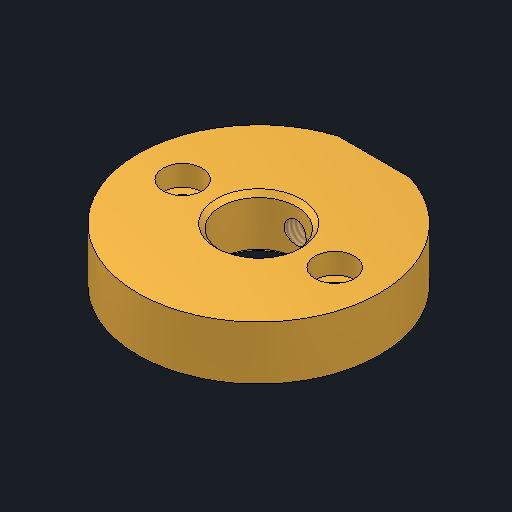
# Autodesk Inventor part: KN-00-02-12
Saved by Autodesk Inventor 2025.2 (Build 292293000, 293)
## iProperties
Created: 2025-04-25
Part Number: KN-00-02-12
Material: CuZn40
Document SubType Name: Modeling
Designer: Kacper Mik
Density: 8.47 g/cm^3
Appearance: Brass - Satin
Author: Kacper Mik
Autodesk Inventor part; units mm, degrees
ref_plane "YZ Plane" through (0, 0, 0) normal (1, 0, 0) x (0, 1, 0)
ref_plane "XZ Plane" through (0, 0, 0) normal (0, 1, 0) x (-1, 0, 0)
ref_plane "XY Plane" through (0, 0, 0) normal (0, 0, 1) x (1, 0, 0)
sketch "Sketch1" plane through (0, 0, 0) normal (0, 1, 0) x (-1, 0, 0)
  circle A0 centre (0, 0) radius 13.5
  dimension "d0" = 27
  constraints: 1 centre point, 1 coincident
  measures "d0" diameter of A0
extrude "Extrusion1" add sketch "Sketch1" along normal blind 6
sketch "Sketch3" plane through (0, 6, 0) normal (0, 1, 0) x (1, 0, 0)
  point P0 (0, 0)
  point P1 (0, 0)
  constraints: 1 coincident
hole "Hole1" at (0, 6, 0) direction (0, -1, 0) diameter 8.5 end through all
sketch "Sketch4" plane through (0, 6, 0) normal (0, 1, 0) x (1, 0, 0)
  point P0 (0, 0)
  point P1 (-8.5, 0)
  point P2 (8.5, 0)
  dimension "d13" = 17
  dimension "d14" = 8.5
  constraints: 2 horizontal alignment
  measures "d13" distance of point (8.5, 0) point (-8.5, 0)
  measures "d14" distance of point (8.5, 0) point (0, 0)
hole "Hole2" at (-8.5, 6, 0) at (8.5, 6, 0) direction (0, -1, 0) diameter 2.4 end through all counterbore diameter 4.4 counterbore depth 2.3 clearance for "Socket Head Cap Screw ISO 4762" size "M2" standard "ISO"
chamfer "Chamfer2" distance 0.5 angle 45 2 edges at (0, 0, -4.25) (0, 6, -4.25)
sketch "Sketch5" plane through (0, 6, 0) normal (0, 1, 0) x (1, 0, 0)
  line L0 (0, 0) -> (4, 12.8938) construction
  circle A0 centre (0, 0) radius 13.5 construction
  line L1 (0, 0) -> (-4, 12.8938) construction
  line L2 (0, 18.9) -> (0, -18.9) construction
  line L3 (4, 12.8938) -> (-4, 12.8938)
  arc A1 (4, 12.8938) -> (-4, 12.8938) centre (0, 0) ccw
  point P0 (0, 13.5)
  dimension "d28" = 8
  constraints: 6 end point, 6 point on circle, 1 centre point, 1 horizontal, 1 point on line, 1 other
  measures "d28" distance of L0.end L1.end
extrude "Extrusion3" cut sketch "Sketch5" against normal through all
sketch "Sketch6" plane through (4, 6, -12.8938) normal (0, 0, -1) x (-1, 0, 0)
  line L0 (8, -6) -> (0, -6) construction
  line L1 (8, 0) -> (8, -6) construction
  line L2 (0, 0) -> (8, 0) construction
  line L3 (0, -6) -> (0, 0) construction
  line L4 (0, 0) -> (8, -6) construction
  point P0 (4, -6)
  point P1 (4, -3)
  constraints: 2 end point, 1 midpoint
hole "Hole3" at (0, 3, -12.8938) direction (0, 0, 1) diameter 2.459 depth 10 tip angle 118 thread size "M3x0.5" class "6H" standard "ISO Metric profile"
chamfer "Chamfer3" distance 0.2 angle 45 1 edges at (0, 1.7705, -12.8938)
equation "\"d14\" = 0.5 * d13"
body "Solid1"
